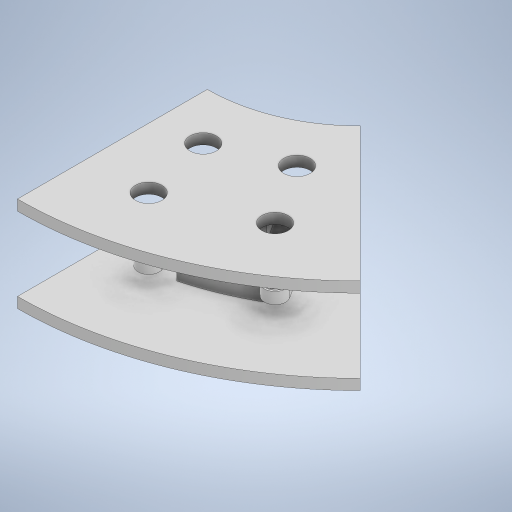
# Autodesk Inventor part: Roller Carousel Part
Saved by Autodesk Inventor 2023 (Build 270158000, 158)
## iProperties
Created: 2022-11-03
Part Number: Roller Carousel Part
Material: Generic
Document SubType Name: Modeling
Designer: cheng
Density: 1 g/cm^3
Appearance: Default
Author: cheng
Autodesk Inventor part; units mm, degrees
ref_plane "YZ Plane" through (0, 0, 0) normal (1, 0, 0) x (0, 1, 0)
ref_plane "XZ Plane" through (0, 0, 0) normal (0, 1, 0) x (-1, 0, 0)
ref_plane "XY Plane" through (0, 0, 0) normal (0, 0, 1) x (1, 0, 0)
sketch "Sketch1" plane through (0, 0, 0) normal (0, 1, 0) x (-1, 0, 0)
  circle A0 centre (0, 0) radius 325
  circle A1 centre (0, 0) radius 145
  line L0 (0, 0) -> (0, 325)
  line L1 (0, 0) -> (-325, 0)
  line L2 (0, 0) -> (-229.8097, 229.8097)
  line L3 (-70.3429, 317.2962) -> (-31.3837, 141.5629)
  circle A2 centre (-57.1401, 257.7421) radius 16 construction
  circle A3 centre (-42.4222, 191.354) radius 16 construction
  line L4 (-174.6224, 274.1022) -> (-77.9084, 122.2918)
  circle A4 centre (-141.8471, 222.6553) radius 16 construction
  circle A5 centre (-105.3107, 165.3047) radius 16 construction
  circle A6 centre (-57.1401, 257.7421) radius 7.5
  circle A7 centre (-42.4222, 191.354) radius 10
  circle A8 centre (-57.1401, 257.7421) radius 10
  circle A9 centre (-42.4222, 191.354) radius 7.5
  circle A10 centre (-105.3107, 165.3047) radius 10
  circle A11 centre (-141.8471, 222.6553) radius 10
  circle A12 centre (-141.8471, 222.6553) radius 7.5
  circle A13 centre (-105.3107, 165.3047) radius 7.5
  line L5 (0, 145) -> (-102.5305, 102.5305)
  line L6 (-51.2652, 123.7652) -> (-73.3756, 177.1443)
  arc A14 (-50.8633, 229.4296) -> (-126.2654, 198.197) centre (25.7109, -62.0716) ccw construction
  line L7 (-89.6264, 216.3774) -> (-100.6301, 242.9426)
  circle A15 centre (0, 0) radius 180
  circle A16 centre (0, 0) radius 280
  circle A17 centre (0, 0) radius 205
  circle A18 centre (0, 0) radius 245
  line L8 (-47.3771, 259.9065) -> (-32.6592, 193.5184)
  line L9 (-66.903, 255.5777) -> (-52.1851, 189.1896)
  line L10 (-133.4132, 228.0283) -> (-96.8768, 170.6777)
  line L11 (-150.281, 217.2823) -> (-113.7446, 159.9317)
  point P0 (-64.4714, 256.1606)
  point P1 (-48.6419, 199.1844)
  point P2 (-49.8272, 259.4071)
  point P3 (-36.1996, 183.5259)
  point P4 (-143.0871, 232.5782)
  point P5 (-96.8416, 159.9873)
  point P6 (-140.6071, 212.7325)
  point P7 (-113.7798, 170.6221)
  point P8 (-62.7465, 236.8288)
  point P9 (-123.0948, 211.8317)
  point P10 (-101.5814, 178.0624)
  point P11 (-54.0803, 197.738)
  point P12 (-135.2287, 204.2993)
  point P13 (-128.0079, 208.8994)
  point P14 (-48.8403, 240.0825)
  point P15 (-40.0077, 201.0582)
  point P16 (-113.8799, 170.4593)
  point P17 (-106.3609, 175.2494)
  point P18 (-57.199, 238.2295)
  point P19 (-48.7116, 199.1286)
  point P20 (-118.4492, 167.3164)
  point P21 (-34.5543, 202.0668)
  point P22 (-43.2206, 241.1576)
  point P23 (-139.9626, 201.0857)
  dimension "d0" = 650
  dimension "d1" = 180
  dimension "d2" = 45
  dimension "d4" = 32
  dimension "d5" = 32
  dimension "d7" = 32
  dimension "d8" = 32
  dimension "d11" = 15
  dimension "d12" = 20
  dimension "d14" = 15
  dimension "d15" = 20
  dimension "d16" = 20
  dimension "d17" = 20
  dimension "d18" = 15
  dimension "d19" = 15
  dimension "d38" = 20
  dimension "d101" = 35
  dimension "d102" = 25
  dimension "d112" = 100
  dimension "d129" = 35
  constraints: 28 point on circle, 24 end point, 19 centre point, 14 coincident, 12 tangent, 6 point on line, 3 line through centre, 3 midpoint, 2 perpendicular, 1 collinear, 1 vertical, 1 other
  measures "d0" diameter of A0
  measures "d1" radial gap between concentric circles of A0 A1
  measures "d2" angle of L2 L0
  measures "d4" diameter of A2
  measures "d5" diameter of A3
  measures "d7" diameter of A4
  measures "d8" diameter of A5
  measures "d11" diameter of A6
  measures "d12" diameter of A7
  measures "d14" diameter of A9
  measures "d15" diameter of A8
  measures "d16" diameter of A10
  measures "d17" diameter of A11
  measures "d18" diameter of A13
  measures "d19" diameter of A12
  measures "d38" angle of L3 L4
  measures "d101" radial gap between concentric circles of A16 A18
  measures "d102" radial gap between concentric circles of A17 A15
  measures "d112" radial gap between concentric circles of A15 A16
  measures "d129" radial gap between concentric circles of A1 A15
extrude "Extrusion1" add sketch "Sketch1" along normal blind 30 contours A8 L3 A6 | L3 A6 A8 | L8 A17 A7 L3 A18 | A18 L3 A8 L8 | A11 L4 A12 | L4 A12 A11 | A8 L3 A18 L9 | L8 A7 A17 | L3 A7 A17 L9 A18 | L11 A11 L4 A18 | A18 L4 A10 A17 L11 | L10 A18 L4 A11 | L9 A17 L10 A18 | A17 L3 A7 | A7 L3 A9 A17 | L3 A17 A7 | A17 A10 L11 | A18 L10 A17 A10 L4 | A17 A7 L9 | A7 A17 L3 A9 | A17 L4 A13 A10 | A10 L4 A17 | A10 A17 L4 | L10 A10 A17 | L4 A13 A17 A10
sketch "Sketch5" plane through (0, 30, 0) normal (0, 1, 0) x (1, 0, 0)
  arc A0 (54.0803, -197.738) -> (101.5814, -178.0624) centre (0, 0) ccw projected
  arc A1 (62.7465, -236.8288) -> (123.0948, -211.8317) centre (0, 0) ccw projected
  arc A2 (62.7465, -236.8288) -> (123.0948, -211.8317) centre (0, 0) ccw projected
  arc A3 (54.0803, -197.738) -> (101.5814, -178.0624) centre (0, 0) ccw projected
  line L0 (62.7465, -236.8288) -> (54.0803, -197.738)
  line L1 (123.0948, -211.8317) -> (101.5814, -178.0624)
  constraints: 4 end point
extrude "Top Pillar" add sketch "Sketch5" along normal blind 20
sketch "Sketch6" plane through (0, 0, 0) normal (0, -1, 0) x (1, 0, 0)
  arc A0 (101.5814, 178.0624) -> (54.0803, 197.738) centre (0, 0) ccw projected
  arc A1 (123.0948, 211.8317) -> (62.7465, 236.8288) centre (0, 0) ccw projected
  line L0 (62.7465, 236.8288) -> (54.0803, 197.738)
  line L1 (96.8768, 170.6777) -> (101.5814, 178.0624) projected
  line L2 (123.0948, 211.8317) -> (101.5814, 178.0624)
  constraints: 4 end point, 1 collinear
extrude "Lower Pillar" add sketch "Sketch6" along normal blind 20
sketch "Sketch7" plane through (0, 50, 0) normal (0, 1, 0) x (1, 0, 0)
  circle A0 centre (0, 0) radius 145
  circle A1 centre (0, 0) radius 325
  arc A2 (52.1851, -189.1896) -> (32.6592, -193.5184) centre (42.4222, -191.354) ccw construction
  arc A3 (113.7446, -159.9317) -> (96.8768, -170.6777) centre (105.3107, -165.3047) ccw construction
  arc A4 (133.4132, -228.0283) -> (150.281, -217.2823) centre (141.8471, -222.6553) ccw construction
  circle A5 centre (57.1401, -257.7421) radius 7.5 construction
  line L0 (60.3204, -250.9498) -> (39.6494, -181.7461) construction
  arc A6 (52.1851, -189.1896) -> (32.6592, -193.5184) centre (42.4222, -191.354) ccw construction
  arc A7 (113.7446, -159.9317) -> (96.8768, -170.6777) centre (105.3107, -165.3047) ccw construction
  line L1 (100.4776, -156.5503) -> (131.4297, -205.569) construction
  arc A8 (133.4132, -228.0283) -> (150.281, -217.2823) centre (141.8471, -222.6553) ccw construction
  circle A9 centre (0, 0) radius 221.6037
  line L2 (49.9849, -216.348) -> (-0.5731, -231.4495) construction
  line L3 (0, 0) -> (229.8097, -229.8097)
  line L4 (0, 0) -> (0, -325)
  line L5 (84.2486, -203.3941) -> (84.8041, -204.7352) construction
  line L6 (0, 0) -> (124.3721, -300.2608) construction
  line L7 (0, 0) -> (325, 0) construction
  line L8 (0, 0) -> (0, -325) construction
  arc A10 (60.5501, -227.0654) -> (117.7441, -203.3748) centre (0, 0) ccw projected
  arc A11 (51.8371, -187.9838) -> (96.2702, -169.579) centre (0, 0) ccw projected
  circle A12 centre (105.3107, -165.3047) radius 7.5 projected
  circle A13 centre (42.4222, -191.354) radius 7.5 projected
  circle A14 centre (141.8471, -222.6553) radius 7.5 projected
  circle A15 centre (57.1401, -257.7421) radius 7.5 projected
  circle A16 centre (105.3107, -165.3047) radius 12.5
  circle A17 centre (141.8471, -222.6553) radius 12.5
  circle A18 centre (57.1401, -257.7421) radius 12.5
  circle A19 centre (42.4222, -191.354) radius 7.5 projected
  circle A20 centre (42.4222, -191.354) radius 12.5
  line L9 (117.7441, -203.3748) -> (96.2702, -169.579) construction
  line L10 (51.8371, -187.9838) -> (60.5501, -227.0654) construction
  line L11 (96.2702, -169.579) -> (60.5501, -227.0654) construction
  line L12 (117.7441, -203.3748) -> (51.8371, -187.9838) construction
  line L13 (80.6528, -194.713) -> (78.8149, -190.2759) construction
  point P0 (102.5305, -102.5305)
  point P1 (0, -145)
  dimension "d82" = 22.5
  dimension "d83" = 22.5
  dimension "d105" = 650
  dimension "d107" = 180
  dimension "d113" = 5
  dimension "d114" = 5
  dimension "d115" = 5
  dimension "d116" = 5
  constraints: 24 end point, 8 point on circle, 7 coincident, 6 centre point, 3 collinear, 2 point on line, 1 horizontal, 1 midpoint, 1 perpendicular, 13 other
  measures "d82" angle of L6 L4
  measures "d83" angle of L6 L3
  measures "d105" diameter of A1
  measures "d107" radial gap between concentric circles of A0 A1
  measures "d113" radial gap between concentric circles of A16 A12
  measures "d114" radial gap between concentric circles of A17 A14
  measures "d115" radial gap between concentric circles of A20 A13
extrude "Top Face" add sketch "Sketch7" along normal blind 10 contours A0 L3 A9 L4 | A9 L3 A1 L4 picked at (123.9054, -138.0996) picked at (179.8075, -201.1178)
sketch "Sketch9" plane through (0, -20, 0) normal (0, -1, 0) x (1, 0, 0)
  arc A0 (229.8097, 229.8097) -> (0, 325) centre (0, 0) ccw projected
  line L0 (229.8097, 229.8097) -> (102.5305, 102.5305) projected
  arc A1 (102.5305, 102.5305) -> (0, 145) centre (0, 0) ccw projected
  line L1 (0, 145) -> (0, 325) projected
extrude "Extrusion5" add sketch "Sketch9" along normal blind 10
sketch "Sketch11" plane through (113.7446, 0, 159.9317) normal (0.8433914, 0, -0.5372996) x (-0.5372996, 0, -0.8433914)
  line L0 (-68, 0) -> (0, 0) projected
  line L1 (-68, 30) -> (0, 30) projected
  line L2 (-48.7958, 20.8803) -> (-94.2979, 20.8803)
  line L3 (-94.2979, 20.8803) -> (-94.2979, 10.8803)
  line L4 (-94.2979, 10.8803) -> (-48.7958, 10.8803)
  line L5 (-48.7958, 10.8803) -> (-48.7958, 20.8803)
  line L6 (-8.756, 20.8803) -> (36.1093, 20.8803)
  line L7 (36.1093, 20.8803) -> (36.1093, 10.8803)
  line L8 (36.1093, 10.8803) -> (-8.756, 10.8803)
  line L9 (-8.756, 10.8803) -> (-8.756, 20.8803)
  line L10 (-94.2979, 20.8803) -> (-48.7958, 10.8803) construction
  line L11 (-94.2979, 10.8803) -> (-48.7958, 20.8803) construction
  line L12 (-71.5469, 15.8803) -> (-86.9159, 15.8803) construction
  line L13 (0, 0) -> (0, 30) projected
  line L14 (-68, 0) -> (-68, 30) projected
  line L15 (-48.7958, 0) -> (-48.7958, 30) projected
  line L16 (-8.756, 0) -> (-8.756, 30) projected
  point P0 (196, 0)
  dimension "d109" = 10
  constraints: 22 end point, 4 parallel, 3 horizontal, 2 collinear, 2 perpendicular, 2 point on line, 1 midpoint
  measures "d109" distance between parallel lines of L4 L2
sketch3d "3D Sketch3"
  arc A0 (102.5305, 50, 102.5305) -> (0, 50, 145) centre (0, 50, 0) ccw
sweep "Sweep3" cut profiles "Sketch11" path "3D Sketch3" contours L14 L2 L5 L4 | L4 L3 L2 L14 | L9 L6 L13 L8 | L13 L6 L7 L8
sketch "Sketch14" plane through (118.4492, 10.8803, 167.3164) normal (0, 1, 0) x (0.8433914, 0, -0.5372996)
  circle A0 centre (-10, 8.6349) radius 17.5
  circle A1 centre (-76.5538, 20.4007) radius 17.5
  point P0 (-10, 204.756)
  dimension "d130" = 35
  dimension "d131" = 35
  constraints: 2 centre point
  measures "d130" diameter of A0
  measures "d131" diameter of A1
extrude "Extrusion8" cut sketch "Sketch14" along normal blind 10
sketch "Sketch15" plane through (105.3107, 10.8803, 165.3047) normal (0, 1, 0) x (0.8433914, 0, -0.5372996)
  circle A0 centre (0, 0) radius 7.5 projected
  circle A1 centre (0, -68) radius 7.5 projected
  circle A2 centre (-90.2933, -52.0789) radius 7.5 projected
  circle A3 centre (-67.0359, 11.8202) radius 7.5 projected
  circle A4 centre (-67.0359, 11.8202) radius 8.5
  circle A5 centre (0, 0) radius 8.5
  circle A6 centre (0, -68) radius 8.5
  circle A7 centre (-90.2933, -52.0789) radius 8.5
  point P0 (0, 196)
  dimension "d134" = 1
  dimension "d135" = 1
  dimension "d136" = 1
  dimension "d137" = 1
  constraints: 4 centre point, 4 coincident
  measures "d134" radial gap between concentric circles of A3 A4
  measures "d135" radial gap between concentric circles of A5 A0
  measures "d136" radial gap between concentric circles of A6 A1
  measures "d137" radial gap between concentric circles of A7 A2
extrude "Extrusion9" add sketch "Sketch15" along normal blind 1
sketch "Sketch16" plane through (42.4222, 20.8803, 191.354) normal (0, -1, 0) x (0.976296, 0, -0.2164396)
  circle A0 centre (0, 0) radius 7.5 projected
  circle A1 centre (67.0359, -11.8202) radius 7.5 projected
  circle A2 centre (0, 0) radius 8.5
  circle A3 centre (67.0359, -11.8202) radius 8.5
  circle A4 centre (90.2933, 52.0789) radius 7.5 projected
  circle A5 centre (0, 68) radius 7.5 projected
  circle A6 centre (90.2933, 52.0789) radius 8.5
  circle A7 centre (0, 68) radius 8.5
  point P0 (0, -196)
  dimension "d140" = 1
  dimension "d141" = 1
  dimension "d142" = 1
  dimension "d143" = 1
  constraints: 4 centre point, 4 coincident
  measures "d140" radial gap between concentric circles of A2 A0
  measures "d141" radial gap between concentric circles of A3 A1
  measures "d142" radial gap between concentric circles of A5 A7
  measures "d143" radial gap between concentric circles of A6 A4
extrude "Extrusion10" add sketch "Sketch16" along normal blind 1
body "Solid1"
